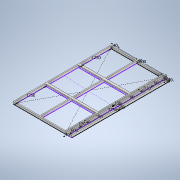
# Autodesk Inventor part: diagrama_cerrajero
Saved by Autodesk Inventor 2021 (Build 250183000, 183)
## iProperties
Created: 2023-12-11
Part Number: diagrama_cerrajero
Material: Generic
Document SubType Name: Modeling
Designer: assman
Density: 1 g/cm^3
Appearance: Default
Author: assman
Autodesk Inventor part; units mm, degrees
ref_plane "YZ Plane" through (0, 0, 0) normal (1, 0, 0) x (0, 1, 0)
ref_plane "XZ Plane" through (0, 0, 0) normal (0, 1, 0) x (-1, 0, 0)
ref_plane "XY Plane" through (0, 0, 0) normal (0, 0, 1) x (1, 0, 0)
sketch "Sketch1" plane through (0, 0, 0) normal (0, 1, 0) x (-1, 0, 0)
  line L0 (1000, 1875) -> (-1000, 1875)
  line L1 (-1000, 1875) -> (-1000, -1875)
  line L2 (-1000, -1875) -> (1000, -1875)
  line L3 (1000, -1875) -> (1000, 1875)
  line L4 (1000, 1875) -> (-1000, -1875) construction
  line L5 (-1000, 1875) -> (1000, -1875) construction
  line L6 (1000, 1875) -> (-1000, 1875)
  line L7 (-1000, 1875) -> (-1000, 1835)
  line L8 (-1000, 1835) -> (1000, 1835)
  line L9 (1000, 1835) -> (1000, 1875)
  line L10 (1000, -1875) -> (-1000, -1875)
  line L11 (-1000, -1875) -> (-1000, -1835)
  line L12 (-1000, -1835) -> (1000, -1835)
  line L13 (1000, -1835) -> (1000, -1875)
  line L14 (-1000, 40) -> (-1000, -40)
  line L15 (1000, -40) -> (1000, 40)
  line L16 (-960, 38.4) -> (1000, -40) construction
  line L17 (1000, 1875) -> (960, 1875)
  line L18 (960, 1835) -> (960, -1835)
  line L19 (960, -1875) -> (1000, -1875)
  line L20 (1000, -1875) -> (1000, 1875)
  line L21 (-1000, 1875) -> (-960, 1875)
  line L22 (-960, 1835) -> (-960, -1835)
  line L23 (-960, -1875) -> (-1000, -1875)
  line L24 (-1000, -1875) -> (-1000, 1875)
  line L25 (20, 1875) -> (-20, 1875)
  line L26 (-20, 1835) -> (-20, -1835)
  line L27 (-20, -1875) -> (20, -1875)
  line L28 (20, -1835) -> (20, 1835)
  line L29 (20, 1875) -> (-20, -1875) construction
  line L30 (-20, 1875) -> (20, -1875) construction
  line L31 (-1000, 1875) -> (-1000, 1275) construction
  line L32 (-1000, -1875) -> (-1000, -1275) construction
  line L33 (-1000, 1275) -> (-1040, 1275)
  line L34 (-1040, 1275) -> (-1040, 1155)
  line L35 (-1040, 1155) -> (-1000, 1155)
  line L36 (-1000, 1155) -> (-1000, 1275)
  line L37 (-1000, -1275) -> (-1040, -1275)
  line L38 (-1040, -1275) -> (-1040, -1155)
  line L39 (-1040, -1155) -> (-1000, -1155)
  line L40 (-1000, -1155) -> (-1000, -1275)
  line L41 (-1000, 60) -> (-1040, 60)
  line L42 (-1040, 60) -> (-1040, -60)
  line L43 (-1040, -60) -> (-1000, -60)
  line L44 (-1000, -60) -> (-1000, 60)
  line L45 (-1040, 1875) -> (-1240, 1875)
  line L46 (-1240, 1875) -> (-1240, -1875)
  line L47 (-1240, -1875) -> (-1040, -1875)
  line L48 (-1040, -1875) -> (-1040, 1875)
  line L49 (-1040, 1875) -> (-1240, 1875)
  line L50 (-1240, 1875) -> (-1240, 1835)
  line L51 (-1240, 1835) -> (-1040, 1835)
  line L52 (-1040, 1835) -> (-1040, 1875)
  line L53 (-1240, 1875) -> (-1200, 1875)
  line L54 (-1200, 1835) -> (-1200, -1835)
  line L55 (-1200, -1875) -> (-1240, -1875)
  line L56 (-1240, -1875) -> (-1240, 1875)
  line L57 (-1040, -1835) -> (-1240, -1835)
  line L58 (-1240, -1835) -> (-1240, -1875)
  line L59 (-1240, -1875) -> (-1040, -1875)
  line L60 (-1040, -1875) -> (-1040, -1835)
  line L61 (-1040, 1875) -> (-1080, 1875)
  line L62 (-1080, 1835) -> (-1080, -1835)
  line L63 (-1080, -1875) -> (-1040, -1875)
  line L64 (-1040, -1875) -> (-1040, 1875)
  line L65 (-1080, 40) -> (-1200, 40)
  line L66 (-1240, 40) -> (-1240, -40)
  line L67 (-1200, -40) -> (-1080, -40)
  line L68 (-1080, -40) -> (-1080, 40)
  line L69 (-998.5851, 1275.1499) -> (-998.5851, 1144.5155) construction
  line L70 (-998.5851, 1144.5155) -> (-1036.0656, 1144.5155) construction
  line L71 (-1036.0656, 1144.5155) -> (-1036.0656, 1275.1499) construction
  line L72 (-1036.0656, 1275.1499) -> (-998.5851, 1275.1499) construction
  line L73 (-1007.8995, 60.5323) -> (-1007.8995, -70.1021) construction
  line L74 (-1007.8995, -70.1021) -> (-1038.0125, -70.1021) construction
  line L75 (-1038.0125, -70.1021) -> (-1038.0125, 60.5323) construction
  line L76 (-1038.0125, 60.5323) -> (-1007.8995, 60.5323) construction
  line L77 (-1037.0125, -1157.0323) -> (-1006.8995, -1157.0323) construction
  line L78 (-1006.8995, -1157.0323) -> (-1006.8995, -1287.6667) construction
  line L79 (-1006.8995, -1287.6667) -> (-1037.0125, -1287.6667) construction
  line L80 (-1037.0125, -1287.6667) -> (-1037.0125, -1157.0323) construction
  line L81 (1000, 1875) -> (1000, 625) construction
  line L82 (1000, -1875) -> (1000, -625) construction
  line L83 (1000, -625) -> (-1000, -625) construction
  line L84 (960, 625) -> (-1000, 625) construction
  line L85 (-960, 665) -> (-960, 585)
  line L86 (960, 585) -> (960, 665)
  line L87 (960, 665) -> (-960, 585) construction
  line L88 (-960, 665) -> (960, 585) construction
  line L89 (-960, -585) -> (-960, -665)
  line L90 (960, -665) -> (960, -585)
  line L91 (960, -585) -> (-960, -665) construction
  line L92 (-960, -585) -> (960, -665) construction
  line L93 (960, 665) -> (20, 665)
  line L94 (-20, 665) -> (-960, 665)
  line L95 (-960, 585) -> (-20, 585)
  line L96 (20, 585) -> (960, 585)
  line L97 (960, -585) -> (20, -585)
  line L98 (-20, -585) -> (-960, -585)
  line L99 (-960, -665) -> (-20, -665)
  line L100 (20, -665) -> (960, -665)
  point P0 (0, 0)
  point P1 (-1000, 0)
  point P2 (-1040, -60)
  point P3 (0, 625)
  point P4 (0, -625)
  dimension "d0" = 2000
  dimension "d1" = 3750
  dimension "d2" = 40
  dimension "d3" = 40
  dimension "d4" = 80
  dimension "d5" = 40
  dimension "d6" = 40
  dimension "d7" = 40
  dimension "d8" = 600
  dimension "d9" = 600
  dimension "d10" = 40
  dimension "d11" = 120
  dimension "d12" = 40
  dimension "d13" = 120
  dimension "d14" = 40
  dimension "d15" = 120
  dimension "d16" = 200
  dimension "d17" = 40
  dimension "d18" = 40
  dimension "d30" = 1250
  dimension "d31" = 1250
  dimension "d32" = 80
  dimension "d33" = 80
  constraints: 178 end point, 47 point on line, 41 parallel, 21 perpendicular, 19 horizontal, 11 midpoint, 6 other
  measures "d0" distance of L2.end L1.end
  measures "d1" distance of L1.end L0.end
  measures "d2" distance of L7.end L6.end
  measures "d3" distance of L10.end L11.end
  measures "d4" distance of L14.end L14.start
  measures "d5" distance of L19.end L19.start
  measures "d6" distance of L23.start L23.end
  measures "d7" distance of L27.end L27.start
  measures "d8" distance of L6.end L31.end
  measures "d9" distance of L23.end L32.end
  measures "d10" distance of L35.end L34.end
  measures "d11" distance of L34.end L33.end
  measures "d12" distance of L38.end L39.end
  measures "d13" distance of L37.end L38.end
  measures "d14" distance of L43.end L42.end
  measures "d15" distance of L42.end L41.end
  measures "d16" distance of L47.end L46.end
  measures "d17" distance of L55.start L55.end
  measures "d18" distance of L63.end L63.start
  measures "d30" distance of L0.start L81.end
  measures "d31" distance of L19.end L82.end
  measures "d32" distance of L85.end L85.start
  measures "d33" distance of L89.end L89.start
extrude "Extrusion1" add sketch "Sketch1" along normal blind 80 contours L3 L8 L1 L0 | L3 L12 L18 L8 | L28 L12 L26 L8 | L3 L2 L1 L12 | L22 L12 L1 L8 | L34 L48 L42 L38 L57 L62 L51 | L51 L46 L45 L48 | L54 L57 L46 L51 | L48 L47 L46 L57
sketch "Sketch2" plane through (0, 80, 0) normal (0, 1, 0) x (1, 0, 0)
  line L0 (960, 40) -> (-1000, 40) construction
  line L1 (-1000, -40) -> (960, -40) construction
  line L2 (1200, 40) -> (1080, 40) construction
  line L3 (1080, -40) -> (1200, -40) construction
  line L4 (1000, -1275) -> (1040, -1275) construction
  line L5 (1040, -1155) -> (1000, -1155) construction
  line L6 (1000, -60) -> (1040, -60) construction
  line L7 (1040, 60) -> (1000, 60) construction
  line L8 (1040, 1155) -> (1000, 1155) construction
  line L9 (1000, 1275) -> (1040, 1275) construction
  line L10 (-960, -1835) -> (-960, 1835) projected
  line L11 (-20, 1835) -> (-20, -1835) projected
  line L12 (-960, -40) -> (-20, -40)
  line L13 (-20, -40) -> (-20, 40)
  line L14 (-20, 40) -> (-960, 40)
  line L15 (-960, 40) -> (-960, -40)
  line L16 (20, -1835) -> (20, 1835) projected
  line L17 (20, -40) -> (960, -40)
  line L18 (960, -40) -> (960, 40)
  line L19 (960, 40) -> (20, 40)
  line L20 (20, 40) -> (20, -40)
  line L21 (1080, -40) -> (1200, -40)
  line L22 (1200, -40) -> (1200, 40)
  line L23 (1200, 40) -> (1080, 40)
  line L24 (1080, 40) -> (1080, -40)
  line L25 (-20, -585) -> (-960, -585) projected
  line L26 (-960, -665) -> (-20, -665) projected
  line L27 (20, -665) -> (960, -665) projected
  line L28 (960, -585) -> (20, -585) projected
  line L29 (20, -1835) -> (20, 1835) projected
  line L30 (960, 1835) -> (960, -1835) projected
  line L31 (-960, 585) -> (-20, 585) projected
  line L32 (-20, 665) -> (-960, 665) projected
  line L33 (20, 585) -> (960, 585) projected
  line L34 (960, 665) -> (20, 665) projected
  point P0 (0, 0)
  constraints: 24 end point, 6 parallel, 5 point on line, 3 horizontal, 3 perpendicular, 1 midpoint, 1 other
sketch "Sketch3" plane through (1000, 0, 1875) normal (1, 0, 0) x (0, 0, -1)
  line L0 (0, 0) -> (3750, 0) construction
  line L1 (3750, 0) -> (3750, 80) construction
  line L2 (0, 80) -> (3750, 80) construction
  line L3 (0, 0) -> (0, 80) construction
  line L4 (0, 0) -> (0, 80) construction
  line L5 (0, 40) -> (3750, 40) construction
  line L6 (0, 80) -> (3750, 80) construction
  line L7 (600, 0) -> (720, 0) construction
  line L8 (720, 0) -> (720, 80) construction
  line L9 (720, 80) -> (600, 80) construction
  line L10 (600, 80) -> (600, 0) construction
  line L11 (1815, 0) -> (1935, 0) construction
  line L12 (1935, 0) -> (1935, 80) construction
  line L13 (1935, 80) -> (1815, 80) construction
  line L14 (1815, 80) -> (1815, 0) construction
  line L15 (3030, 0) -> (3150, 0) construction
  line L16 (3150, 0) -> (3150, 80) construction
  line L17 (3150, 80) -> (3030, 80) construction
  line L18 (3030, 80) -> (3030, 0) construction
  point P0 (1875, 0)
  point P1 (660, 40)
  point P2 (1878.8319, 40)
  point P3 (3090, 40)
  constraints: 26 end point, 6 parallel, 6 point on line, 3 horizontal, 3 perpendicular, 2 midpoint
ref_plane "Work Plane1" through (1000, 40, 1215) normal (0, 0, 1) x (1, 0, 0)
ref_plane "Work Plane2" through (1000, 40, -3.8319) normal (0, 0, 1) x (1, 0, 0)
ref_plane "Work Plane3" through (1000, 40, -1215) normal (0, 0, 1) x (1, 0, 0)
sketch "Sketch4" plane through (1000, 40, 1215) normal (0, 0, 1) x (1, 0, 0)
  circle A0 centre (20, 20) radius 20
  line L0 (40, -40) -> (40, 40) projected
  line L1 (-2000, 40) -> (0, 40) construction
  line L2 (0, 40) -> (40, 40) construction
  point P0 (-1000, -40)
  dimension "d23" = 40
  constraints: 2 end point, 2 tangent, 1 centre point
  measures "d23" diameter of A0
sketch "Sketch5" plane through (1000, 40, -3.8319) normal (0, 0, 1) x (1, 0, 0)
  point P0 (-1000, -40)
sketch "Sketch6" plane through (1000, 40, -3.8319) normal (0, 0, 1) x (1, 0, 0)
  circle A0 centre (20, 20) radius 20 projected
  point P0 (-1000, -40)
sketch "Sketch7" plane through (1000, 40, -1215) normal (0, 0, 1) x (1, 0, 0)
  circle A0 centre (20, 20) radius 20 projected
  point P0 (-1000, -40)
extrude "Extrusion3" add sketch "Sketch4" along normal mid plane 120
extrude "Extrusion4" add sketch "Sketch6" along normal mid plane 120
extrude "Extrusion5" add sketch "Sketch7" along normal mid plane 120
extrude "Extrusion6" add sketch "Sketch2" against normal blind 40 contours L10 L25 L11 L26 | L10 L32 L11 L31 | L16 L28 L30 L27 | L16 L34 L30 L33
body "Solid1"
